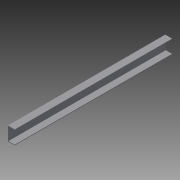
# Autodesk Inventor part: Part56061 Aluminum Channel 3in x 1.5in
Saved by Autodesk Inventor 2015 (Build 190159000, 159)
## iProperties
Created: 2016-01-16
Part Number: Part56061 Aluminum Channel 3in x 1.5in
Material: Generic
Document SubType Name: Modeling
Designer: sethbattis
Density: 1 g/cm^3
Appearance: Default
Author: sethbattis
Autodesk Inventor part; units mm, degrees
ref_plane "YZ Plane" through (0, 0, 0) normal (1, 0, 0) x (0, 1, 0)
ref_plane "XZ Plane" through (0, 0, 0) normal (0, 1, 0) x (-1, 0, 0)
ref_plane "XY Plane" through (0, 0, 0) normal (0, 0, 1) x (1, 0, 0)
sketch "Sketch1" plane through (0, 0, 0) normal (0, 0, 1) x (1, 0, 0)
  line L0 (0, 0) -> (0, 76.2)
  line L1 (0, 76.2) -> (38.1, 76.2)
  line L2 (38.1, 76.2) -> (38.1, 72.898)
  line L3 (38.1, 72.898) -> (3.302, 72.898)
  line L4 (3.302, 72.898) -> (3.302, 3.302)
  line L5 (3.302, 3.302) -> (38.1, 3.302)
  line L6 (38.1, 3.302) -> (38.1, 0)
  line L7 (38.1, 0) -> (0, 0)
  dimension "d0" = 76.2
  dimension "d1" = 38.1
  dimension "d2" = 3.302
  dimension "d3" = 3.302
  constraints: 16 end point, 7 perpendicular, 2 equal length, 1 horizontal
  measures "d0" distance of L0.start L0.end
  measures "d1" distance of L0.end L1.end
  measures "d2" distance of L1.end L2.end
  measures "d3" distance between parallel lines of L4 L0
extrude "Extrusion1" add sketch "Sketch1" along normal blind 869.95
body "Solid1"
